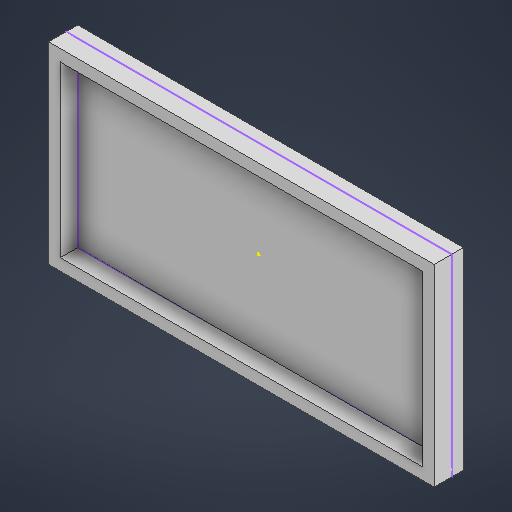
# Autodesk Inventor part: Deksel laser
Saved by Autodesk Inventor 2026.2 (Build 302298000, 298)
## iProperties
Created: 2026-05-05
Part Number: Deksel laser
Material: Generic
Document SubType Name: Modeling
Designer: Gameb
Density: 1 g/cm^3
Appearance: Default
Author: Gameb
Autodesk Inventor part; units mm, degrees
ref_plane "YZ Plane" through (0, 0, 0) normal (1, 0, 0) x (0, 1, 0)
ref_plane "XZ Plane" through (0, 0, 0) normal (0, 1, 0) x (-1, 0, 0)
ref_plane "XY Plane" through (0, 0, 0) normal (0, 0, 1) x (1, 0, 0)
sketch "Sketch1" plane through (0, 0, 0) normal (0, 0, 1) x (1, 0, 0)
  line L0 (-62, 0) -> (-62, 9.0726)
  line L1 (-62, 0) -> (-62, 29)
  line L2 (-62, 29) -> (-62, -29)
  line L3 (-62, -29) -> (62, -29)
  line L4 (62, -29) -> (62, 29)
  line L5 (62, 29) -> (-62, 29)
  line L6 (-62, 33) -> (-66, 33)
  line L7 (-66, 33) -> (-66, -29)
  line L8 (-66, -29) -> (-66, -33)
  line L9 (-66, -33) -> (-62, -33)
  line L10 (-62, -33) -> (62, -33)
  line L11 (62, -33) -> (66, -33)
  line L12 (66, -33) -> (66, -29)
  line L13 (66, -29) -> (66, 29)
  line L14 (66, 29) -> (66, 33)
  line L15 (62, 33) -> (66, 33)
  line L16 (62, 33) -> (-62, 33)
  point P0 (0, 0)
  constraints: 34 end point, 9 point on line, 6 perpendicular, 1 collinear
extrude "Extrusion1" add sketch "Sketch1" against normal blind 4 contours L0 L1 L5 L4 L3 L2 | L16 L15 L14 L13 L12 L11 L10 L9 L8 L7 L6
extrude "Extrusion2" add sketch "Sketch1" along normal blind 6
body "Solid1"
